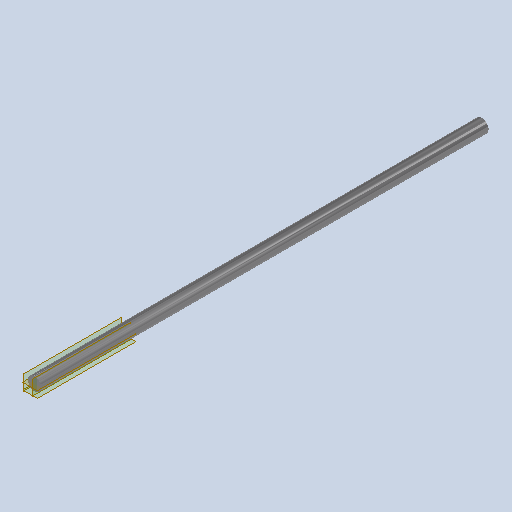
# Autodesk Inventor part: 13-505
Saved by Autodesk Inventor 2022 (Build 260153000, 153)
## iProperties
Created: 2004-09-20
Part Number: 13-505
Material: Acciaio dolce
Document SubType Name: Modeling
Designer: Chapin
Manufacturer: Standard
Standards Organization: Custom
Mass: 44.4473 g
Surface Area: 38.2646 cm^2
Volume: 5.65487 cm^3
Density: 7.86 g/cm^3
Appearance: Cromo
d4: 0,000 mm
d5: 0,000 mm
d7: 0,000 mm
d9: 0,000 mm
d10: 0,000 mm
d11: 0,000 mm
Author: Chapin
Autodesk Inventor part; units mm, degrees
ref_plane "YZ Plane" through (0, 0, 0) normal (1, 0, 0) x (0, 1, 0)
ref_plane "XZ Plane" through (0, 0, 0) normal (0, 1, 0) x (-1, 0, 0)
ref_plane "XY Plane" through (0, 0, 0) normal (0, 0, 1) x (1, 0, 0)
sketch "Sketch1" plane through (0, 0, 0) normal (0, 0, 1) x (1, 0, 0)
  circle A0 centre (0, 0) radius 3
  dimension "d0" = 6
  constraints: 1 centre point, 1 coincident
  measures "d0" diameter of A0
extrude "Extrusion1" add sketch "Sketch1" against normal blind 200
ref_plane "Side1" through (1, 0, 0) normal (-1, 0, 0) x (0, -1, 0)
ref_plane "T-Slot1" through (0, 0, 0) normal (0, 1, 0) x (0, 0, -1)
ref_plane "Side2" through (-3, 0, 0) normal (-1, 0, 0) x (0, -1, 0)
ref_plane "Side3" through (0, -3, 0) normal (0, -1, 0) x (1, 0, 0)
equation "\"d1\" = Ex_Length"
equation "\"Ex_Length\" = 200"
